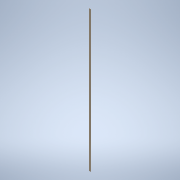
# Autodesk Inventor part: SP57V1 Felpa Detectores
Saved by Autodesk Inventor 2021.2 (Build 252289000, 289)
## iProperties
Created: 2026-10-05
Part Number: SP57V1 Felpa Detectores
Material: Fabric
Document SubType Name: Modeling
Designer: nelso
Density: 0.9 g/cm^3
Appearance: Smooth - Off-White
Author: nelso
Autodesk Inventor part; units mm, degrees
ref_plane "YZ Plane" through (0, 0, 0) normal (1, 0, 0) x (0, 1, 0)
ref_plane "XZ Plane" through (0, 0, 0) normal (0, 1, 0) x (-1, 0, 0)
ref_plane "XY Plane" through (0, 0, 0) normal (0, 0, 1) x (1, 0, 0)
sketch "Sketch1" plane through (0, 0, 0) normal (0, 1, 0) x (-1, 0, 0)
  line L0 (7, 565) -> (-7, 565)
  line L1 (-7, 565) -> (-7, -565)
  line L2 (-7, -565) -> (7, -565)
  line L3 (7, -565) -> (7, 565)
  line L4 (7, 565) -> (-7, -565) construction
  line L5 (-7, 565) -> (7, -565) construction
  point P0 (0, 0)
  dimension "d0" = 14
  dimension "d1" = 1130
  constraints: 12 end point, 2 midpoint, 2 parallel, 1 horizontal, 1 perpendicular
  measures "d0" distance of L2.end L1.end
  measures "d1" distance of L1.end L0.end
extrude "Extrusion1" add sketch "Sketch1" along normal blind 2
body "Solid1"
